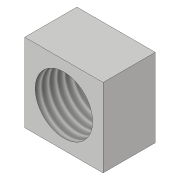
# Autodesk Inventor part: bolt1
Saved by Autodesk Inventor 2019 (Build 230136000, 136)
## iProperties
Created: 2019-10-07
Part Number: bolt1
Material: Generic
Document SubType Name: Modeling
Designer: Admin
Density: 1 g/cm^3
Appearance: Default
Author: Admin
Autodesk Inventor part; units mm, degrees
ref_plane "YZ Plane" through (0, 0, 0) normal (1, 0, 0) x (0, 1, 0)
ref_plane "XZ Plane" through (0, 0, 0) normal (0, 1, 0) x (-1, 0, 0)
ref_plane "XY Plane" through (0, 0, 0) normal (0, 0, 1) x (1, 0, 0)
sketch "Sketch1" plane through (0, 0, 0) normal (0, 0, 1) x (1, 0, 0)
  point P0 (0, 0)
sketch "Sketch2" plane through (0, 0, 0) normal (0, 0, 1) x (1, 0, 0)
  line L0 (0, 0) -> (15, 0)
  line L1 (15, 0) -> (15, 15)
  line L2 (15, 15) -> (0, 15)
  line L3 (0, 15) -> (0, 0)
  line L4 (0, 7.9375) -> (15.875, 7.9375)
  line L5 (7.9375, 15) -> (7.9375, 0)
  dimension "d0" = 15
  dimension "d1" = 15
  constraints: 12 end point, 3 perpendicular, 3 point on line, 2 parallel, 1 horizontal
  measures "d0" distance of L2.end L1.end
  measures "d1" distance of L1.end L0.end
extrude "Extrusion1" add sketch "Sketch2" along normal blind 10
sketch "Sketch3" plane through (0, 0, 10) normal (0, 0, 1) x (1, 0, 0)
  line L0 (0, 14.9966) -> (7.5, 15)
  line L1 (15, 15) -> (0, 15) projected
  line L2 (0.0034, 7.4661) -> (15, 7.2509)
  arc A0 (7.5017, 0) -> (7.5, 15) centre (-22407.2052, 4.9864) ccw
  circle A1 centre (7.5021, 7.5) radius 5.5
  point P0 (0, 0)
  dimension "d4" = 11
  constraints: 4 end point, 3 point on circle, 2 centre point, 1 midpoint, 1 point on line
  measures "d4" diameter of A1
extrude "Extrusion2" cut sketch "Sketch3" along normal through all both and the other way through all
thread "Thread1" size "M11x1.5" class "6H" standard "ANSI Metric M Profile" full length
body "Solid1"
